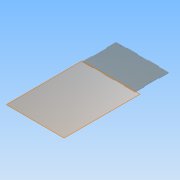
# Autodesk Inventor part: back part
Saved by Autodesk Inventor 2017 (Build 210142000, 142)
## iProperties
Part Number: back part
Material: Типовые
Document SubType Name: Modeling
Designer: Max
Mass: 385.563 g
Surface Area: 1987.62 cm^2
Volume: 385.563 cm^3
Density: 1 g/cm^3
Appearance: Поликарбонат — дымчатый
Author: Max
Autodesk Inventor part; units mm, degrees
(part 1 of 2)
ref_plane "YZ Plane" through (0, 0, 0) normal (1, 0, 0) x (0, 1, 0)
ref_plane "XZ Plane" through (0, 0, 0) normal (0, 1, 0) x (-1, 0, 0)
ref_plane "XY Plane" through (0, 0, 0) normal (0, 0, 1) x (1, 0, 0)
ref_plane "РабПлоскость1" through (0, 0, 0) normal (0, 0, 1) x (1, 0, 0)
sketch "Эскиз1" plane through (0, 0, 0) normal (0, 0, 1) x (1, 0, 0)
  line L0 (1.5, 784) -> (1.5, 779)
  line L1 (1.5, 779) -> (2.8, 779)
  line L2 (2.8, 779) -> (2.8, 776.55)
  line L3 (2.8, 776.55) -> (1.5, 776.55)
  line L4 (1.5, 776.55) -> (1.5, 775.5)
  line L5 (1.5, 775.5) -> (-1.5, 775.5)
  line L6 (-1.5, 775.5) -> (-1.5, 776.55)
  line L7 (-1.5, 776.55) -> (-2.8, 776.55)
  line L8 (-2.8, 776.55) -> (-2.8, 779)
  line L9 (-2.8, 779) -> (-1.5, 779)
  line L10 (-1.5, 779) -> (-1.5, 784)
  line L11 (-1.5, 784) -> (-39.3, 784)
  line L12 (-39.3, 784) -> (-39.3, 788)
  line L13 (-39.3, 788) -> (-116.7, 788)
  line L14 (-116.7, 788) -> (-116.7, 784)
  line L15 (-116.7, 784) -> (-154.35, 784)
  line L16 (-154.35, 784) -> (-154.35, 779)
  line L17 (-154.35, 779) -> (-153.05, 779)
  line L18 (-153.05, 779) -> (-153.05, 776.55)
  line L19 (-153.05, 776.55) -> (-154.35, 776.55)
  line L20 (-154.35, 776.55) -> (-154.35, 775.5)
  line L21 (-154.35, 775.5) -> (-157.35, 775.5)
  line L22 (-157.35, 775.5) -> (-157.35, 776.55)
  line L23 (-157.35, 776.55) -> (-158.65, 776.55)
  line L24 (-158.65, 776.55) -> (-158.65, 779)
  line L25 (-158.65, 779) -> (-157.35, 779)
  line L26 (-157.35, 779) -> (-157.35, 784)
  line L27 (-157.35, 784) -> (-195, 784)
  line L28 (-195, 784) -> (-195, 26) projected
  line L29 (-195, 26) -> (-145, 26) projected
  line L30 (-145, 26) -> (-145, 324) projected
  line L31 (-145, 324) -> (-125, 344) projected
  line L32 (-125, 344) -> (125, 344) projected
  line L33 (125, 344) -> (145, 324) projected
  line L34 (145, 324) -> (145, 26) projected
  line L35 (145, 26) -> (195, 26) projected
  line L36 (195, 26) -> (195, 784) projected
  line L37 (195, 784) -> (157.35, 784)
  line L38 (157.35, 784) -> (157.35, 779)
  line L39 (157.35, 779) -> (158.65, 779)
  line L40 (158.65, 779) -> (158.65, 776.55)
  line L41 (158.65, 776.55) -> (157.35, 776.55)
  line L42 (157.35, 776.55) -> (157.35, 775.5)
  line L43 (157.35, 775.5) -> (154.35, 775.5)
  line L44 (154.35, 775.5) -> (154.35, 776.55)
  line L45 (154.35, 776.55) -> (153.05, 776.55)
  line L46 (153.05, 776.55) -> (153.05, 779)
  line L47 (153.05, 779) -> (154.35, 779)
  line L48 (154.35, 779) -> (154.35, 784)
  line L49 (154.35, 784) -> (116.7, 784)
  line L50 (116.7, 784) -> (116.7, 788)
  line L51 (116.7, 788) -> (39.3, 788)
  line L52 (39.3, 788) -> (39.3, 784)
  line L53 (39.3, 784) -> (1.5, 784)
  circle A0 centre (181, 376) radius 5 projected
  circle A1 centre (-181, 376) radius 5 projected
  circle A2 centre (-179, 349) radius 5 projected
  circle A3 centre (179, 349) radius 5 projected
  line L54 (-131.1498, 477.7505) -> (-131.1498, 487.2505) projected
  arc A4 (-130.8998, 487.5005) -> (-131.1498, 487.2505) centre (-130.8998, 487.2505) ccw projected
  line L55 (-130.8998, 487.5005) -> (-108.8998, 487.5005) projected
  arc A5 (-108.6498, 487.2505) -> (-108.8998, 487.5005) centre (-108.8998, 487.2505) ccw projected
  line L56 (-108.6498, 487.2505) -> (-108.6498, 477.7505) projected
  arc A6 (-108.8998, 477.5005) -> (-108.6498, 477.7505) centre (-108.8998, 477.7505) ccw projected
  line L57 (-108.8998, 477.5005) -> (-130.8998, 477.5005) projected
  arc A7 (-131.1498, 477.7505) -> (-130.8998, 477.5005) centre (-130.8998, 477.7505) ccw projected
  spline S0 degree 2 poles (-108.6858, 451.2309) (-108.6858, 452.7138) (-109.7069, 454.8289) (-110.7523, 455.4245) knots 0 0 0 1 2 2 2 projected
  spline S1 degree 2 poles (-110.7523, 455.4245) (-111.5181, 455.8378) (-113.1955, 455.9229) (-114.3625, 455.9229) knots 0 0 0 1 2 2 2 projected
  line L58 (-114.3625, 455.9229) -> (-118.2036, 455.9229) projected
  line L59 (-118.2036, 455.9229) -> (-118.2036, 458.7187) projected
  line L60 (-118.2036, 458.7187) -> (-113.5602, 458.7187) projected
  spline S2 degree 2 poles (-113.5602, 458.7187) (-111.98, 458.7187) (-109.2207, 458.3176) (-108.0051, 457.5396) knots 0 0 0 1 2 2 2 projected
  spline S3 degree 2 poles (-108.0051, 457.5396) (-106.5343, 456.5915) (-104.8203, 453.3825) (-104.8203, 451.2066) knots 0 0 0 1 2 2 2 projected
  spline S4 degree 2 poles (-104.8203, 451.2066) (-104.8203, 449.1036) (-106.6558, 445.7973) (-108.0537, 444.91) knots 0 0 0 1 2 2 2 projected
  spline S5 degree 2 poles (-108.0537, 444.91) (-109.2206, 444.1563) (-111.9678, 443.7186) (-113.5116, 443.7187) knots 0 0 0 1 2 2 2 projected
  line L61 (-113.5116, 443.7187) -> (-118.2036, 443.7187) projected
  line L62 (-118.2036, 443.7187) -> (-118.2036, 446.5267) projected
  line L63 (-118.2036, 446.5267) -> (-114.3625, 446.5267) projected
  spline S6 degree 2 poles (-114.3625, 446.5267) (-113.0983, 446.5267) (-111.36, 446.6118) (-110.5699, 447.1101) knots 0 0 0 1 2 2 2 projected
  spline S7 degree 2 poles (-110.5699, 447.1101) (-109.6461, 447.6936) (-108.6858, 449.7479) (-108.6858, 451.2309) knots 0 0 0 1 2 2 2 projected
  line L64 (-122.3998, 476.0005) -> (-122.3998, 477.0005) projected
  line L65 (-122.3998, 477.0005) -> (-117.3998, 477.0005) projected
  line L66 (-117.3998, 477.0005) -> (-117.3998, 476.0005) projected
  line L67 (-117.3998, 476.0005) -> (-115.3998, 476.0005) projected
  line L68 (-115.3998, 476.0005) -> (-115.3998, 473.0005) projected
  spline S8 degree 2 poles (-115.3998, 473.0005) (-116.5248, 471.7942) (-117.6498, 473.0005) knots -0.936411 -0.936411 -0.936411 0 0 0 weights 1 1.154701 1 projected
  spline S9 degree 2 poles (-117.6498, 473.0005) (-119.8998, 471.7942) (-122.1498, 473.0005) knots -0.936411 -0.936411 -0.936411 0 0 0 weights 1 1.154701 1 projected
  spline S10 degree 2 poles (-122.1498, 473.0005) (-123.2748, 471.7942) (-124.3998, 473.0005) knots 0 0 0 0.936411 0.936411 0.936411 weights 1 1.154701 1 projected
  line L69 (-124.3998, 473.0005) -> (-124.3998, 476.0005) projected
  line L70 (-124.3998, 476.0005) -> (-122.3998, 476.0005) projected
  line L71 (-119.5248, 468.5774) -> (-120.2748, 468.5774) projected
  line L72 (-120.2748, 468.5774) -> (-123.3048, 471.8264) projected
  spline S11 degree 3 poles (-123.3048, 471.8264) (-123.2674, 471.8256) (-123.1923, 471.8269) (-123.099, 471.836) (-123.0063, 471.8503) (-122.9329, 471.866) (-122.8423, 471.8907) (-122.7708, 471.9142) (-122.6828, 471.9483) (-122.6134, 471.9792) (-122.528, 472.0219) (-122.4606, 472.0595) (-122.3773, 472.1105) (-122.3114, 472.1544) (-122.2297, 472.2133) (-122.1486, 472.2762) (-122.0839, 472.3308) (-122.0515, 472.3592) knots 0.459691 0.459691 0.459691 0.459691 0.491589 0.523488 0.539437 0.571336 0.587285 0.619184 0.635133 0.667032 0.682981 0.71488 0.730829 0.762728 0.778677 0.810576 0.842474 0.842474 0.842474 0.842474 projected
  spline S12 degree 3 poles (-122.0515, 472.3592) (-121.923, 472.2982) (-121.6714, 472.1878) (-121.3667, 472.0767) (-121.0671, 471.9849) (-120.8308, 471.9266) (-120.538, 471.872) (-120.3054, 471.843) (-120.0156, 471.8248) (-119.7841, 471.8248) (-119.4942, 471.843) (-119.2616, 471.872) (-118.9103, 471.9375) (-118.4363, 472.064) (-118.0051, 472.2371) (-117.7481, 472.3592) knots 0.060134 0.060134 0.060134 0.060134 0.128146 0.196158 0.230164 0.298176 0.332182 0.400194 0.4342 0.502211 0.536217 0.604229 0.638235 0.740253 0.876277 0.876277 0.876277 0.876277 projected
  spline S13 degree 3 poles (-117.7481, 472.3592) (-117.7158, 472.3308) (-117.6511, 472.2762) (-117.5699, 472.2133) (-117.4882, 472.1544) (-117.4223, 472.1105) (-117.3391, 472.0595) (-117.2717, 472.0219) (-117.1862, 471.9792) (-117.1169, 471.9483) (-117.0288, 471.9142) (-116.9573, 471.8907) (-116.8667, 471.866) (-116.7933, 471.8503) (-116.7007, 471.836) (-116.6073, 471.8269) (-116.5323, 471.8256) (-116.4948, 471.8264) knots 0.093937 0.093937 0.093937 0.093937 0.125835 0.157734 0.173683 0.205582 0.221531 0.25343 0.269379 0.301278 0.317227 0.349126 0.365075 0.396974 0.412923 0.444822 0.47672 0.47672 0.47672 0.47672 projected
  line L73 (-116.4948, 471.8264) -> (-119.5248, 468.5774) projected
  line L74 (-114.4354, 446.5678) -> (-118.2036, 446.5678) projected
  line L75 (-118.2036, 446.5678) -> (-118.2036, 455.9186) projected
  line L76 (-118.2036, 455.9186) -> (-114.4354, 455.9186) projected
  line L77 (-114.4354, 455.9186) -> (-114.4354, 446.5678) projected
  arc A8 (-119.3998, 461.3273) -> (-120.8998, 462.8273) centre (-120.8998, 461.3273) ccw projected
  line L78 (-119.3998, 461.3273) -> (-119.3998, 460.8273) projected
  line L79 (-119.3998, 460.8273) -> (-120.3998, 460.8273) projected
  line L80 (-120.3998, 460.8273) -> (-120.3998, 461.3273) projected
  arc A9 (-120.3998, 461.3273) -> (-120.8998, 461.8273) centre (-120.8998, 461.3273) ccw projected
  line L81 (-120.8998, 461.8273) -> (-127.3998, 461.8273) projected
  arc A10 (-127.3998, 464.8273) -> (-127.3998, 461.8273) centre (-127.3998, 463.3273) ccw projected
  line L82 (-127.3998, 464.8273) -> (-112.3998, 464.8273) projected
  arc A11 (-112.3998, 464.8273) -> (-112.3998, 465.8273) centre (-112.3998, 465.3273) ccw projected
  line L83 (-112.3998, 465.8273) -> (-118.8998, 465.8273) projected
  arc A12 (-120.3998, 467.3273) -> (-118.8998, 465.8273) centre (-118.8998, 467.3273) ccw projected
  line L84 (-120.3998, 467.3273) -> (-120.3998, 467.8273) projected
  line L85 (-120.3998, 467.8273) -> (-119.3998, 467.8273) projected
  line L86 (-119.3998, 467.8273) -> (-119.3998, 467.3273) projected
  arc A13 (-119.3998, 467.3273) -> (-118.8998, 466.8273) centre (-118.8998, 467.3273) ccw projected
  line L87 (-118.8998, 466.8273) -> (-112.3998, 466.8273) projected
  arc A14 (-112.3998, 463.8273) -> (-112.3998, 466.8273) centre (-112.3998, 465.3273) ccw projected
  line L88 (-112.3998, 463.8273) -> (-127.3998, 463.8273) projected
  arc A15 (-127.3998, 463.8273) -> (-127.3998, 462.8273) centre (-127.3998, 463.3273) ccw projected
  line L89 (-127.3998, 462.8273) -> (-120.8998, 462.8273) projected
  spline S14 degree 2 poles (-122.6526, 458.1231) (-121.8868, 457.649) (-121.121, 456.1904) (-121.121, 455.2787) knots 0 0 0 1 2 2 2 projected
  spline S15 degree 2 poles (-121.121, 455.2787) (-121.121, 453.9902) (-122.604, 452.0696) (-123.8195, 451.79) knots 0 0 0 1 2 2 2 projected
  line L90 (-123.8195, 451.79) -> (-123.8195, 451.6442) projected
  spline S16 degree 2 poles (-123.8195, 451.6442) (-123.2847, 451.5712) (-122.2636, 451.1822) (-121.7774, 450.7446) knots 0 0 0 1 2 2 2 projected
  spline S17 degree 2 poles (-121.7774, 450.7446) (-121.3276, 450.3557) (-120.732, 449.1158) (-120.732, 448.2649) knots 0 0 0 1 2 2 2 projected
  spline S18 degree 2 poles (-120.732, 448.2649) (-120.732, 447.1587) (-121.5464, 445.3476) (-122.3365, 444.7155) knots 0 0 0 1 2 2 2 projected
  spline S19 degree 2 poles (-122.3365, 444.7155) (-123.1267, 444.0834) (-125.2782, 443.4027) (-126.822, 443.4027) knots 0 0 0 1 2 2 2 projected
  spline S20 degree 2 poles (-126.822, 443.4027) (-128.5724, 443.4026) (-131.0764, 443.9861) (-131.8665, 444.3508) knots 0 0 0 1 2 2 2 projected
  line L91 (-131.8665, 444.3508) -> (-131.8665, 447.6085) projected
  line L92 (-131.8665, 447.6085) -> (-131.5019, 447.6085) projected
  spline S21 degree 2 poles (-131.5019, 447.6085) (-130.6753, 447.0858) (-128.4508, 446.3079) (-127.527, 446.3079) knots 0 0 0 1 2 2 2 projected
  spline S22 degree 2 poles (-127.527, 446.3079) (-126.98, 446.3079) (-125.7036, 446.5024) (-125.266, 446.8184) knots 0 0 0 1 2 2 2 projected
  spline S23 degree 2 poles (-125.266, 446.8184) (-124.9257, 447.0737) (-124.5124, 447.8151) (-124.5124, 448.4837) knots 0 0 0 1 2 2 2 projected
  spline S24 degree 2 poles (-124.5124, 448.4837) (-124.5124, 449.1523) (-125.0959, 449.8694) (-125.5821, 450.0396) knots 0 0 0 1 2 2 2 projected
  spline S25 degree 2 poles (-125.5821, 450.0396) (-126.0683, 450.2098) (-127.4176, 450.2463) (-127.9403, 450.2463) knots 0 0 0 1 2 2 2 projected
  line L93 (-127.9403, 450.2463) -> (-128.5845, 450.2463) projected
  line L94 (-128.5845, 450.2463) -> (-128.5845, 452.884) projected
  line L95 (-128.5845, 452.884) -> (-127.9889, 452.884) projected
  spline S26 degree 2 poles (-127.9889, 452.884) (-127.3082, 452.884) (-126.1534, 453.0056) (-125.7523, 453.1879) knots 0 0 0 1 2 2 2 projected
  spline S27 degree 2 poles (-125.7523, 453.1879) (-125.3511, 453.3824) (-124.9014, 454.0631) (-124.9014, 454.6466) knots 0 0 0 1 2 2 2 projected
  spline S28 degree 2 poles (-124.9014, 454.6466) (-124.9014, 455.1085) (-125.3268, 455.6798) (-125.6307, 455.8378) knots 0 0 0 1 2 2 2 projected
  spline S29 degree 2 poles (-125.6307, 455.8378) (-125.9954, 456.0202) (-126.9678, 456.1417) (-127.3082, 456.1417) knots 0 0 0 1 2 2 2 projected
  spline S30 degree 2 poles (-127.3082, 456.1417) (-127.8552, 456.1417) (-129.01, 455.8864) (-129.5448, 455.6798) knots 0 0 0 1 2 2 2 projected
  spline S31 degree 2 poles (-129.5448, 455.6798) (-129.9703, 455.5218) (-130.7084, 455.1139) (-130.8976, 455.0047) knots 0 0 0 1 1.597943 1.597943 1.597943 projected
  line L96 (-130.8976, 455.0047) -> (-131.3629, 454.8775) projected
  line L97 (-131.3629, 454.8775) -> (-131.4289, 454.8775) projected
  line L98 (-131.4289, 454.8775) -> (-131.4289, 458.0866) projected
  spline S32 degree 2 poles (-131.4289, 458.0866) (-130.651, 458.4148) (-128.0254, 459.0348) (-126.6518, 459.0348) knots 0 0 0 1 2 2 2 projected
  spline S33 degree 2 poles (-126.6518, 459.0348) (-125.3147, 459.0348) (-123.3455, 458.5729) (-122.6526, 458.1231) knots 0 0 0 1 2 2 2 projected
  line L99 (-119.9951, 430.5006) -> (-119.9951, 437.0006) projected
  arc A16 (-119.9951, 437.0006) -> (-119.9952, 437.0006) centre (-119.8998, 464.5005) ccw projected
  line L100 (-119.9952, 437.0006) -> (-119.9952, 430.5006) projected
  arc A17 (-124.3998, 430.7996) -> (-119.9952, 430.5006) centre (-119.8998, 464.5005) ccw projected
  arc A18 (-126.1498, 434.137) -> (-124.3998, 430.7996) centre (-112.6193, 439.1042) ccw projected
  arc A19 (-136.9506, 438.6109) -> (-126.1498, 434.137) centre (-119.8998, 464.5005) ccw projected
  arc A20 (-140.548, 437.4884) -> (-136.9506, 438.6109) centre (-143.0058, 451.6907) ccw projected
  arc A21 (-146.9119, 443.8523) -> (-140.548, 437.4884) centre (-119.8998, 464.5005) ccw projected
  arc A22 (-145.7894, 447.4497) -> (-146.9119, 443.8523) centre (-132.7096, 441.3945) ccw projected
  arc A23 (-150.2632, 458.2505) -> (-145.7894, 447.4497) centre (-119.8998, 464.5005) ccw projected
  arc A24 (-153.6007, 460.0005) -> (-150.2632, 458.2505) centre (-145.2961, 471.781) ccw projected
  arc A25 (-153.6007, 469.0005) -> (-153.6007, 460.0005) centre (-119.8998, 464.5005) ccw projected
  arc A26 (-150.2632, 470.7505) -> (-153.6007, 469.0005) centre (-145.2961, 457.2199) ccw projected
  arc A27 (-145.7894, 481.5512) -> (-150.2632, 470.7505) centre (-119.8998, 464.5005) ccw projected
  arc A28 (-146.9119, 485.1486) -> (-145.7894, 481.5512) centre (-132.7096, 487.6064) ccw projected
  arc A29 (-140.548, 491.5126) -> (-146.9119, 485.1486) centre (-119.8998, 464.5005) ccw projected
  arc A30 (-136.9506, 490.3901) -> (-140.548, 491.5126) centre (-143.0058, 477.3102) ccw projected
  arc A31 (-126.1498, 494.8639) -> (-136.9506, 490.3901) centre (-119.8998, 464.5005) ccw projected
  arc A32 (-124.3998, 498.2014) -> (-126.1498, 494.8639) centre (-112.6193, 489.8967) ccw projected
  arc A33 (-115.3998, 498.2014) -> (-124.3998, 498.2014) centre (-119.8998, 464.5005) ccw projected
  arc A34 (-113.6498, 494.8639) -> (-115.3998, 498.2014) centre (-127.1803, 489.8967) ccw projected
  arc A35 (-102.8491, 490.3901) -> (-113.6498, 494.8639) centre (-119.8998, 464.5005) ccw projected
  arc A36 (-99.2517, 491.5126) -> (-102.8491, 490.3901) centre (-96.7939, 477.3102) ccw projected
  arc A37 (-92.8877, 485.1486) -> (-99.2517, 491.5126) centre (-119.8998, 464.5005) ccw projected
  arc A38 (-94.0102, 481.5512) -> (-92.8877, 485.1486) centre (-107.0901, 487.6064) ccw projected
  arc A39 (-89.5364, 470.7505) -> (-94.0102, 481.5512) centre (-119.8998, 464.5005) ccw projected
  arc A40 (-86.1989, 469.0005) -> (-89.5364, 470.7505) centre (-94.5036, 457.2199) ccw projected
  arc A41 (-86.1989, 460.0005) -> (-86.1989, 469.0005) centre (-119.8998, 464.5005) ccw projected
  arc A42 (-89.5364, 458.2505) -> (-86.1989, 460.0005) centre (-94.5036, 471.781) ccw projected
  arc A43 (-94.0102, 447.4497) -> (-89.5364, 458.2505) centre (-119.8998, 464.5005) ccw projected
  arc A44 (-92.8877, 443.8523) -> (-94.0102, 447.4497) centre (-107.0901, 441.3945) ccw projected
  arc A45 (-99.2517, 437.4884) -> (-92.8877, 443.8523) centre (-119.8998, 464.5005) ccw projected
  arc A46 (-102.8491, 438.6109) -> (-99.2517, 437.4884) centre (-96.7939, 451.6907) ccw projected
  arc A47 (-113.6498, 434.137) -> (-102.8491, 438.6109) centre (-119.8998, 464.5005) ccw projected
  arc A48 (-115.3998, 430.7996) -> (-113.6498, 434.137) centre (-127.1803, 439.1042) ccw projected
  arc A49 (-119.9951, 430.5006) -> (-115.3998, 430.7996) centre (-119.8998, 464.5005) ccw projected
  circle A50 centre (1, 464) radius 20.6 projected
  circle A51 centre (179.5, 40) radius 2 projected
  circle A52 centre (-179.5, 79.5) radius 2 projected
  circle A53 centre (-179.5, 337) radius 2 projected
  circle A54 centre (179.5, 337) radius 2 projected
  circle A55 centre (179.5, 255) radius 2.875 projected
  circle A56 centre (-179.5, 308) radius 2 projected
  circle A57 centre (-179.5, 40) radius 2 projected
  circle A58 centre (-158.75, 122) radius 1.5 projected
  circle A59 centre (-158.75, 254) radius 1.5 projected
  circle A60 centre (-158.75, 284) radius 1.5 projected
  circle A61 centre (-158.75, 92) radius 1.5 projected
  circle A62 centre (150.2671, 178.4783) radius 1.5 projected
  line L101 (116.2244, 383.4424) -> (116.2244, 380.5646) projected
  line L102 (116.2244, 380.5646) -> (110.4314, 380.5646) projected
  line L103 (110.4314, 380.5646) -> (110.1311, 378.6127) projected
  spline S34 degree 2 poles (110.1311, 378.6127) (110.7316, 378.888) (111.9078, 379.1758) (112.4833, 379.1758) knots 0 0 0 1 2 2 2 projected
  spline S35 degree 2 poles (112.4833, 379.1758) (114.4227, 379.1758) (116.85, 376.811) (116.85, 375.0218) knots 0 0 0 1 2 2 2 projected
  spline S36 degree 2 poles (116.85, 375.0218) (116.85, 373.7706) (115.5988, 371.4433) (113.3091, 370.2172) (111.5199, 370.2172) knots 0 0 0 1 2 3 3 3 projected
  spline S37 degree 2 poles (111.5199, 370.2172) (110.2312, 370.2172) (108.4044, 370.7051) (107.1157, 371.6686) (106.3149, 372.8947) (106.0521, 373.8081) knots 0 0 0 1 2 3 4 4 4 projected
  line L104 (106.0521, 373.8081) -> (109.7057, 374.2085) projected
  spline S38 degree 2 poles (109.7057, 374.2085) (109.8433, 373.3327) (110.8067, 372.4193) (111.4824, 372.4193) knots 0 0 0 1 2 2 2 projected
  spline S39 degree 2 poles (111.4824, 372.4193) (112.2331, 372.4193) (113.209, 373.5579) (113.209, 374.6965) knots 0 0 0 1 2 2 2 projected
  spline S40 degree 2 poles (113.209, 374.6965) (113.209, 375.8601) (112.2206, 376.9361) (111.4073, 376.9361) knots 0 0 0 1 2 2 2 projected
  spline S41 degree 2 poles (111.4073, 376.9361) (110.8818, 376.9361) (110.3938, 376.6734) knots 0 0 0 1 1 1 projected
  spline S42 degree 2 poles (110.3938, 376.6734) (110.0435, 376.4982) (109.6056, 376.0102) knots 0 0 0 1 1 1 projected
  line L105 (109.6056, 376.0102) -> (106.5276, 376.4481) projected
  line L106 (106.5276, 376.4481) -> (107.6662, 383.4424) projected
  line L107 (107.6662, 383.4424) -> (116.2244, 383.4424) projected
  spline S43 degree 2 poles (77.5998, 374.9842) (77.7249, 374.0458) (78.1003, 373.5579) knots 0 0 0 1 1 1 projected
  spline S44 degree 2 poles (78.1003, 373.5579) (78.7259, 372.7696) (79.8895, 372.7696) knots 0 0 0 1 1 1 projected
  spline S45 degree 2 poles (79.8895, 372.7696) (80.7403, 372.7696) (81.6787, 373.5829) (81.6787, 374.1084) knots 0 0 0 1 2 2 2 projected
  spline S46 degree 2 poles (81.6787, 374.1084) (81.6787, 374.6089) (81.2283, 375.0093) knots 0 0 0 1 1 1 projected
  spline S47 degree 2 poles (81.2283, 375.0093) (80.7904, 375.4096) (79.1763, 375.7725) knots 0 0 0 1 1 1 projected
  spline S48 degree 2 poles (79.1763, 375.7725) (76.5237, 376.3606) (75.3977, 377.349) knots 0 0 0 1 1 1 projected
  spline S49 degree 2 poles (75.3977, 377.349) (74.2591, 378.3375) (74.2591, 379.8639) knots 0 0 0 1 1 1 projected
  spline S50 degree 2 poles (74.2591, 379.8639) (74.2591, 380.8649) (75.4227, 382.6416) (77.7624, 383.6676) (79.7894, 383.6676) knots 0 0 0 1 2 3 3 3 projected
  spline S51 degree 2 poles (79.7894, 383.6676) (82.2918, 383.6676) (84.9068, 381.8158) (85.157, 379.7889) knots 0 0 0 1 2 2 2 projected
  line L108 (85.157, 379.7889) -> (81.3659, 379.5636) projected
  spline S52 degree 2 poles (81.3659, 379.5636) (81.2158, 380.4395) (80.2398, 381.2403) (79.389, 381.2403) knots 0 0 0 1 2 2 2 projected
  spline S53 degree 2 poles (79.389, 381.2403) (78.6883, 381.2403) (77.9751, 380.6522) (77.9751, 380.2143) knots 0 0 0 1 2 2 2 projected
  spline S54 degree 2 poles (77.9751, 380.2143) (77.9751, 379.914) (78.2754, 379.6637) knots 0 0 0 1 1 1 projected
  spline S55 degree 2 poles (78.2754, 379.6637) (78.5632, 379.401) (79.6267, 379.1883) knots 0 0 0 1 1 1 projected
  spline S56 degree 2 poles (79.6267, 379.1883) (82.2668, 378.6127) (84.544, 377.4491) (85.5825, 375.735) (85.5825, 374.6714) knots 0 0 0 1 2 3 3 3 projected
  spline S57 degree 2 poles (85.5825, 374.6714) (85.5825, 373.4202) (84.1936, 371.3057) (81.7162, 370.2172) (79.8144, 370.2172) knots 0 0 0 1 2 3 3 3 projected
  spline S58 degree 2 poles (79.8144, 370.2172) (76.4987, 370.2172) (73.9338, 372.7696) (73.7711, 374.7465) knots 0 0 0 1 2 2 2 projected
  line L109 (73.7711, 374.7465) -> (77.5998, 374.9842) projected
  spline S59 degree 2 poles (65.5507, 383.6676) (68.7913, 383.6676) (72.3072, 380.1767) (72.3072, 377.0362) knots 0 0 0 1 2 2 2 projected
  spline S60 degree 2 poles (72.3072, 377.0362) (72.3072, 374.759) (70.7682, 371.8437) (67.8654, 370.2172) (65.7008, 370.2172) knots 0 0 0 1 2 3 3 3 projected
  spline S61 degree 2 poles (65.7008, 370.2172) (63.5112, 370.2172) (60.621, 371.6185) (58.8317, 374.6589) (58.8317, 376.9361) knots 0 0 0 1 2 3 3 3 projected
  spline S62 degree 2 poles (58.8317, 376.9361) (58.8317, 380.1142) (62.3852, 383.6676) (65.5507, 383.6676) knots 0 0 0 1 2 2 2 projected
  line L110 (35.6094, 377.8495) -> (41.8154, 377.8495) projected
  line L111 (41.8154, 377.8495) -> (41.8154, 372.3192) projected
  spline S63 degree 2 poles (41.8154, 372.3192) (40.0262, 371.093) (37.286, 370.2172) (35.4092, 370.2172) knots 0 0 0 1 2 2 2 projected
  spline S64 degree 2 poles (35.4092, 370.2172) (33.0945, 370.2172) (30.1667, 371.7937) (28.5651, 374.9217) (28.5651, 376.9486) knots 0 0 0 1 2 3 3 3 projected
  spline S65 degree 2 poles (28.5651, 376.9486) (28.5651, 379.0757) (30.3168, 382.2162) (32.0185, 383.042) knots 0 0 0 1 2 2 2 projected
  spline S66 degree 2 poles (32.0185, 383.042) (33.3447, 383.6676) (35.5719, 383.6676) knots 0 0 0 1 1 1 projected
  spline S67 degree 2 poles (35.5719, 383.6676) (37.7365, 383.6676) (39.876, 382.8918) (41.2899, 381.2403) (41.6402, 379.9891) knots 0 0 0 1 2 3 3 3 projected
  line L112 (41.6402, 379.9891) -> (37.7615, 379.2884) projected
  spline S68 degree 2 poles (37.7615, 379.2884) (37.5238, 380.0266) (36.3726, 380.8148) (35.4843, 380.8148) knots 0 0 0 1 2 2 2 projected
  spline S69 degree 2 poles (35.4843, 380.8148) (34.1705, 380.8148) (32.594, 378.9756) (32.594, 376.9862) knots 0 0 0 1 2 2 2 projected
  spline S70 degree 2 poles (32.594, 376.9862) (32.594, 374.8841) (34.183, 373.0699) (35.6094, 373.0699) knots 0 0 0 1 2 2 2 projected
  spline S71 degree 2 poles (35.6094, 373.0699) (36.2851, 373.0699) (37.5112, 373.4578) (38.2995, 373.9332) knots 0 0 0 1 2 2 2 projected
  line L113 (38.2995, 373.9332) -> (38.2995, 375.1469) projected
  line L114 (38.2995, 375.1469) -> (35.6094, 375.1469) projected
  line L115 (35.6094, 375.1469) -> (35.6094, 377.8495) projected
  line L116 (8.9212, 383.4424) -> (15.6152, 383.4424) projected
  spline S72 degree 2 poles (15.6152, 383.4424) (17.467, 383.4424) (19.4439, 382.8043) (20.645, 381.0776) (20.645, 379.8389) knots 0 0 0 1 2 3 3 3 projected
  spline S73 degree 2 poles (20.645, 379.8389) (20.645, 378.7504) (19.7191, 377.1864) (18.9184, 376.6984) knots 0 0 0 1 2 2 2 projected
  spline S74 degree 2 poles (18.9184, 376.6984) (18.4054, 376.3856) (17.5045, 376.1854) knots 0 0 0 1 1 1 projected
  spline S75 degree 2 poles (17.5045, 376.1854) (18.2177, 375.9477) (18.5555, 375.7099) knots 0 0 0 1 1 1 projected
  spline S76 degree 2 poles (18.5555, 375.7099) (18.7682, 375.5473) (19.6065, 374.4963) (19.7567, 374.2085) knots 0 0 0 1 2 2 2 projected
  line L117 (19.7567, 374.2085) -> (21.696, 370.4424) projected
  line L118 (21.696, 370.4424) -> (17.1542, 370.4424) projected
  line L119 (17.1542, 370.4424) -> (15.0146, 374.4212) projected
  spline S77 degree 2 poles (15.0146, 374.4212) (14.6142, 375.1844) (14.3014, 375.4222) knots 0 0 0 1 1 1 projected
  spline S78 degree 2 poles (14.3014, 375.4222) (13.8635, 375.7225) (13.313, 375.7225) knots 0 0 0 1 1 1 projected
  line L120 (13.313, 375.7225) -> (12.9626, 375.7225) projected
  line L121 (12.9626, 375.7225) -> (12.9626, 370.4424) projected
  line L122 (12.9626, 370.4424) -> (8.9212, 370.4424) projected
  line L123 (8.9212, 370.4424) -> (8.9212, 383.4424) projected
  line L124 (-1.8516, 372.5944) -> (-2.4897, 370.4424) projected
  line L125 (-2.4897, 370.4424) -> (-6.5937, 370.4424) projected
  line L126 (-6.5937, 370.4424) -> (-1.7015, 383.4424) projected
  line L127 (-1.7015, 383.4424) -> (2.6903, 383.4424) projected
  line L128 (2.6903, 383.4424) -> (7.5699, 370.4424) projected
  line L129 (7.5699, 370.4424) -> (3.3659, 370.4424) projected
  line L130 (3.3659, 370.4424) -> (2.7153, 372.5944) projected
  line L131 (2.7153, 372.5944) -> (-1.8516, 372.5944) projected
  spline S79 degree 2 poles (-25.0114, 383.4424) (-23.1346, 383.4424) (-21.1201, 381.5781) (-21.1201, 380.2018) knots 0 0 0 1 2 2 2 projected
  spline S80 degree 2 poles (-21.1201, 380.2018) (-21.1201, 379.0507) (-21.8333, 378.2249) knots 0 0 0 1 1 1 projected
  spline S81 degree 2 poles (-21.8333, 378.2249) (-22.3213, 377.6743) (-23.2472, 377.349) knots 0 0 0 1 1 1 projected
  spline S82 degree 2 poles (-23.2472, 377.349) (-21.8458, 377.0112) (-20.5196, 375.3721) (-20.5196, 374.1334) knots 0 0 0 1 2 2 2 projected
  spline S83 degree 2 poles (-20.5196, 374.1334) (-20.5196, 373.1325) (-21.458, 371.5184) (-22.2712, 371.043) knots 0 0 0 1 2 2 2 projected
  spline S84 degree 2 poles (-22.2712, 371.043) (-22.7842, 370.7552) (-23.7977, 370.6175) knots 0 0 0 1 1 1 projected
  spline S85 degree 2 poles (-23.7977, 370.6175) (-25.1615, 370.4424) (-25.5994, 370.4424) knots 0 0 0 1 1 1 projected
  line L132 (-25.5994, 370.4424) -> (-32.5311, 370.4424) projected
  line L133 (-32.5311, 370.4424) -> (-32.5311, 383.4424) projected
  line L134 (-32.5311, 383.4424) -> (-25.0114, 383.4424) projected
  line L135 (-65.0999, 383.4424) -> (-60.1952, 376.248) projected
  line L136 (-60.1952, 376.248) -> (-60.1952, 383.4424) projected
  line L137 (-60.1952, 383.4424) -> (-56.4041, 383.4424) projected
  line L138 (-56.4041, 383.4424) -> (-56.4041, 370.4424) projected
  line L139 (-56.4041, 370.4424) -> (-60.1952, 370.4424) projected
  line L140 (-60.1952, 370.4424) -> (-65.0749, 377.5993) projected
  line L141 (-65.0749, 377.5993) -> (-65.0749, 370.4424) projected
  line L142 (-65.0749, 370.4424) -> (-68.8535, 370.4424) projected
  line L143 (-68.8535, 370.4424) -> (-68.8535, 383.4424) projected
  line L144 (-68.8535, 383.4424) -> (-65.0999, 383.4424) projected
  line L145 (-86.9334, 383.4424) -> (-84.3184, 379.0632) projected
  line L146 (-84.3184, 379.0632) -> (-81.6909, 383.4424) projected
  line L147 (-81.6909, 383.4424) -> (-77.2491, 383.4424) projected
  line L148 (-77.2491, 383.4424) -> (-82.304, 375.8851) projected
  line L149 (-82.304, 375.8851) -> (-82.304, 370.4424) projected
  line L150 (-82.304, 370.4424) -> (-86.3328, 370.4424) projected
  line L151 (-86.3328, 370.4424) -> (-86.3328, 375.8851) projected
  line L152 (-86.3328, 375.8851) -> (-91.4002, 383.4424) projected
  line L153 (-91.4002, 383.4424) -> (-86.9334, 383.4424) projected
  line L154 (-104.3877, 383.4424) -> (-104.3877, 380.6522) projected
  line L155 (-104.3877, 380.6522) -> (-110.2684, 380.6522) projected
  line L156 (-110.2684, 380.6522) -> (-110.2684, 378.3875) projected
  line L157 (-110.2684, 378.3875) -> (-105.251, 378.3875) projected
  line L158 (-105.251, 378.3875) -> (-105.251, 375.76) projected
  line L159 (-105.251, 375.76) -> (-110.2684, 375.76) projected
  line L160 (-110.2684, 375.76) -> (-110.2684, 370.4424) projected
  line L161 (-110.2684, 370.4424) -> (-114.3097, 370.4424) projected
  line L162 (-114.3097, 370.4424) -> (-114.3097, 383.4424) projected
  line L163 (-114.3097, 383.4424) -> (-104.3877, 383.4424) projected
  line L164 (-98.1942, 383.4424) -> (-98.1942, 373.6455) projected
  line L165 (-98.1942, 373.6455) -> (-91.9257, 373.6455) projected
  line L166 (-91.9257, 373.6455) -> (-91.9257, 370.4424) projected
  line L167 (-91.9257, 370.4424) -> (-102.2106, 370.4424) projected
  line L168 (-102.2106, 370.4424) -> (-102.2106, 383.4424) projected
  line L169 (-102.2106, 383.4424) -> (-98.1942, 383.4424) projected
  line L170 (-71.7563, 383.4424) -> (-71.7563, 370.4424) projected
  line L171 (-71.7563, 370.4424) -> (-75.7852, 370.4424) projected
  line L172 (-75.7852, 370.4424) -> (-75.7852, 383.4424) projected
  line L173 (-75.7852, 383.4424) -> (-71.7563, 383.4424) projected
  line L174 (-47.1827, 377.8495) -> (-40.9767, 377.8495) projected
  line L175 (-40.9767, 377.8495) -> (-40.9767, 372.3192) projected
  spline S86 degree 2 poles (-40.9767, 372.3192) (-42.7659, 371.093) (-45.5061, 370.2172) (-47.3829, 370.2172) knots 0 0 0 1 2 2 2 projected
  spline S87 degree 2 poles (-47.3829, 370.2172) (-49.6976, 370.2172) (-52.6254, 371.7937) (-54.227, 374.9217) (-54.227, 376.9486) knots 0 0 0 1 2 3 3 3 projected
  spline S88 degree 2 poles (-54.227, 376.9486) (-54.227, 379.0757) (-52.4753, 382.2162) (-50.7736, 383.042) knots 0 0 0 1 2 2 2 projected
  spline S89 degree 2 poles (-50.7736, 383.042) (-49.4474, 383.6676) (-47.2202, 383.6676) knots 0 0 0 1 1 1 projected
  spline S90 degree 2 poles (-47.2202, 383.6676) (-45.0557, 383.6676) (-42.9161, 382.8918) (-41.5022, 381.2403) (-41.1519, 379.9891) knots 0 0 0 1 2 3 3 3 projected
  line L176 (-41.1519, 379.9891) -> (-45.0306, 379.2884) projected
  spline S91 degree 2 poles (-45.0306, 379.2884) (-45.2684, 380.0266) (-46.4195, 380.8148) (-47.3078, 380.8148) knots 0 0 0 1 2 2 2 projected
  spline S92 degree 2 poles (-47.3078, 380.8148) (-48.6216, 380.8148) (-50.1981, 378.9756) (-50.1981, 376.9862) knots 0 0 0 1 2 2 2 projected
  spline S93 degree 2 poles (-50.1981, 376.9862) (-50.1981, 374.8841) (-48.6091, 373.0699) (-47.1827, 373.0699) knots 0 0 0 1 2 2 2 projected
  spline S94 degree 2 poles (-47.1827, 373.0699) (-46.507, 373.0699) (-45.2809, 373.4578) (-44.4926, 373.9332) knots 0 0 0 1 2 2 2 projected
  line L177 (-44.4926, 373.9332) -> (-44.4926, 375.1469) projected
  line L178 (-44.4926, 375.1469) -> (-47.1827, 375.1469) projected
  line L179 (-47.1827, 375.1469) -> (-47.1827, 377.8495) projected
  line L180 (-7.6447, 383.4424) -> (-7.6447, 380.6647) projected
  line L181 (-7.6447, 380.6647) -> (-14.3762, 380.6647) projected
  line L182 (-14.3762, 380.6647) -> (-14.3762, 378.6002) projected
  line L183 (-14.3762, 378.6002) -> (-8.1326, 378.6002) projected
  line L184 (-8.1326, 378.6002) -> (-8.1326, 375.9477) projected
  line L185 (-8.1326, 375.9477) -> (-14.3762, 375.9477) projected
  line L186 (-14.3762, 375.9477) -> (-14.3762, 373.3827) projected
  line L187 (-14.3762, 373.3827) -> (-7.4445, 373.3827) projected
  line L188 (-7.4445, 373.3827) -> (-7.4445, 370.4424) projected
  line L189 (-7.4445, 370.4424) -> (-18.405, 370.4424) projected
  line L190 (-18.405, 370.4424) -> (-18.405, 383.4424) projected
  line L191 (-18.405, 383.4424) -> (-7.6447, 383.4424) projected
  line L192 (48.234, 383.4424) -> (48.234, 378.888) projected
  line L193 (48.234, 378.888) -> (52.6258, 378.888) projected
  line L194 (52.6258, 378.888) -> (52.6258, 383.4424) projected
  line L195 (52.6258, 383.4424) -> (56.6672, 383.4424) projected
  line L196 (56.6672, 383.4424) -> (56.6672, 370.4424) projected
  line L197 (56.6672, 370.4424) -> (52.6258, 370.4424) projected
  line L198 (52.6258, 370.4424) -> (52.6258, 375.6974) projected
  line L199 (52.6258, 375.6974) -> (48.234, 375.6974) projected
  line L200 (48.234, 375.6974) -> (48.234, 370.4424) projected
  line L201 (48.234, 370.4424) -> (44.2177, 370.4424) projected
  line L202 (44.2177, 370.4424) -> (44.2177, 383.4424) projected
  line L203 (44.2177, 383.4424) -> (48.234, 383.4424) projected
  line L204 (98.9078, 383.4424) -> (98.9078, 380.2268) projected
  line L205 (98.9078, 380.2268) -> (94.8038, 380.2268) projected
  line L206 (94.8038, 380.2268) -> (94.8038, 370.4424) projected
  line L207 (94.8038, 370.4424) -> (90.7875, 370.4424) projected
  line L208 (90.7875, 370.4424) -> (90.7875, 380.2268) projected
  line L209 (90.7875, 380.2268) -> (86.6835, 380.2268) projected
  line L210 (86.6835, 380.2268) -> (86.6835, 383.4424) projected
  line L211 (86.6835, 383.4424) -> (98.9078, 383.4424) projected
  line L212 (1.5, 534) -> (1.5, 529) projected
  line L213 (1.5, 529) -> (2.8, 529) projected
  line L214 (2.8, 529) -> (2.8, 526.55) projected
  line L215 (2.8, 526.55) -> (1.5, 526.55) projected
  line L216 (1.5, 526.55) -> (1.5, 525.5) projected
  line L217 (1.5, 525.5) -> (-1.5, 525.5) projected
  line L218 (-1.5, 525.5) -> (-1.5, 526.55) projected
  line L219 (-1.5, 526.55) -> (-2.8, 526.55) projected
  line L220 (-2.8, 526.55) -> (-2.8, 529) projected
  line L221 (-2.8, 529) -> (-1.5, 529) projected
  line L222 (-1.5, 529) -> (-1.5, 534) projected
  line L223 (-1.5, 534) -> (-39.3, 534) projected
  line L224 (-39.3, 534) -> (-39.3, 538) projected
  line L225 (-39.3, 538) -> (-116.7, 538) projected
  line L226 (-116.7, 538) -> (-116.7, 534) projected
  line L227 (-116.7, 534) -> (-154.35, 534) projected
  line L228 (-154.35, 534) -> (-154.35, 529) projected
  line L229 (-154.35, 529) -> (-153.05, 529) projected
  line L230 (-153.05, 529) -> (-153.05, 526.55) projected
  line L231 (-153.05, 526.55) -> (-154.35, 526.55) projected
  line L232 (-154.35, 526.55) -> (-154.35, 525.5) projected
  line L233 (-154.35, 525.5) -> (-157.35, 525.5) projected
  line L234 (-157.35, 525.5) -> (-157.35, 526.55) projected
  line L235 (-157.35, 526.55) -> (-158.65, 526.55) projected
  line L236 (-158.65, 526.55) -> (-158.65, 529) projected
  line L237 (-158.65, 529) -> (-157.35, 529) projected
  line L238 (-157.35, 529) -> (-157.35, 534) projected
  line L239 (-157.35, 534) -> (-195, 534) projected
  line L240 (-195, 534) -> (-195, 26) projected
  line L241 (-195, 26) -> (-145, 26) projected
  line L242 (-145, 26) -> (-145, 324) projected
  line L243 (-145, 324) -> (-125, 344) projected
  line L244 (-125, 344) -> (125, 344) projected
  line L245 (125, 344) -> (145, 324) projected
  line L246 (145, 324) -> (145, 26) projected
  line L247 (145, 26) -> (195, 26) projected
  line L248 (195, 26) -> (195, 534) projected
  line L249 (195, 534) -> (157.35, 534) projected
  line L250 (157.35, 534) -> (157.35, 529) projected
  line L251 (157.35, 529) -> (158.65, 529) projected
  line L252 (158.65, 529) -> (158.65, 526.55) projected
  line L253 (158.65, 526.55) -> (157.35, 526.55) projected
  line L254 (157.35, 526.55) -> (157.35, 525.5) projected
  line L255 (157.35, 525.5) -> (154.35, 525.5) projected
  line L256 (154.35, 525.5) -> (154.35, 526.55) projected
  line L257 (154.35, 526.55) -> (153.05, 526.55) projected
  line L258 (153.05, 526.55) -> (153.05, 529) projected
  line L259 (153.05, 529) -> (154.35, 529) projected
  line L260 (154.35, 529) -> (154.35, 534) projected
  line L261 (154.35, 534) -> (116.7, 534) projected
  line L262 (116.7, 534) -> (116.7, 538) projected
  line L263 (116.7, 538) -> (39.3, 538) projected
  line L264 (39.3, 538) -> (39.3, 534) projected
  line L265 (39.3, 534) -> (1.5, 534) projected
  circle A63 centre (181, 376) radius 5 projected
  circle A64 centre (-181, 376) radius 5 projected
  circle A65 centre (-179, 349) radius 5 projected
  circle A66 centre (179, 349) radius 5 projected
  line L266 (-131.1498, 477.7505) -> (-131.1498, 487.2505) projected
  arc A67 (-130.8998, 487.5005) -> (-131.1498, 487.2505) centre (-130.8998, 487.2505) ccw projected
  line L267 (-130.8998, 487.5005) -> (-108.8998, 487.5005) projected
  arc A68 (-108.6498, 487.2505) -> (-108.8998, 487.5005) centre (-108.8998, 487.2505) ccw projected
  line L268 (-108.6498, 487.2505) -> (-108.6498, 477.7505) projected
  arc A69 (-108.8998, 477.5005) -> (-108.6498, 477.7505) centre (-108.8998, 477.7505) ccw projected
  line L269 (-108.8998, 477.5005) -> (-130.8998, 477.5005) projected
  arc A70 (-131.1498, 477.7505) -> (-130.8998, 477.5005) centre (-130.8998, 477.7505) ccw projected
  spline S95 degree 2 poles (-108.6858, 451.2309) (-108.6858, 452.7138) (-109.7069, 454.8289) (-110.7523, 455.4245) knots 0 0 0 1 2 2 2 projected
  spline S96 degree 2 poles (-110.7523, 455.4245) (-111.5181, 455.8378) (-113.1955, 455.9229) (-114.3625, 455.9229) knots 0 0 0 1 2 2 2 projected
  line L270 (-114.3625, 455.9229) -> (-118.2036, 455.9229) projected
  line L271 (-118.2036, 455.9229) -> (-118.2036, 458.7187) projected
  line L272 (-118.2036, 458.7187) -> (-113.5602, 458.7187) projected
  spline S97 degree 2 poles (-113.5602, 458.7187) (-111.98, 458.7187) (-109.2207, 458.3176) (-108.0051, 457.5396) knots 0 0 0 1 2 2 2 projected
  spline S98 degree 2 poles (-108.0051, 457.5396) (-106.5343, 456.5915) (-104.8203, 453.3825) (-104.8203, 451.2066) knots 0 0 0 1 2 2 2 projected
  spline S99 degree 2 poles (-104.8203, 451.2066) (-104.8203, 449.1036) (-106.6558, 445.7973) (-108.0537, 444.91) knots 0 0 0 1 2 2 2 projected
  spline S100 degree 2 poles (-108.0537, 444.91) (-109.2206, 444.1563) (-111.9678, 443.7186) (-113.5116, 443.7187) knots 0 0 0 1 2 2 2 projected
  line L273 (-113.5116, 443.7187) -> (-118.2036, 443.7187) projected
  line L274 (-118.2036, 443.7187) -> (-118.2036, 446.5267) projected
  line L275 (-118.2036, 446.5267) -> (-114.3625, 446.5267) projected
  spline S101 degree 2 poles (-114.3625, 446.5267) (-113.0983, 446.5267) (-111.36, 446.6118) (-110.5699, 447.1101) knots 0 0 0 1 2 2 2 projected
  spline S102 degree 2 poles (-110.5699, 447.1101) (-109.6461, 447.6936) (-108.6858, 449.7479) (-108.6858, 451.2309) knots 0 0 0 1 2 2 2 projected
  line L276 (-122.3998, 476.0005) -> (-122.3998, 477.0005) projected
  line L277 (-122.3998, 477.0005) -> (-117.3998, 477.0005) projected
  line L278 (-117.3998, 477.0005) -> (-117.3998, 476.0005) projected
  line L279 (-117.3998, 476.0005) -> (-115.3998, 476.0005) projected
  line L280 (-115.3998, 476.0005) -> (-115.3998, 473.0005) projected
  spline S103 degree 2 poles (-115.3998, 473.0005) (-116.5248, 471.7942) (-117.6498, 473.0005) knots -0.936411 -0.936411 -0.936411 0 0 0 weights 1 1.154701 1 projected
  spline S104 degree 2 poles (-117.6498, 473.0005) (-119.8998, 471.7942) (-122.1498, 473.0005) knots -0.936411 -0.936411 -0.936411 0 0 0 weights 1 1.154701 1 projected
  spline S105 degree 2 poles (-122.1498, 473.0005) (-123.2748, 471.7942) (-124.3998, 473.0005) knots 0 0 0 0.936411 0.936411 0.936411 weights 1 1.154701 1 projected
  line L281 (-124.3998, 473.0005) -> (-124.3998, 476.0005) projected
  line L282 (-124.3998, 476.0005) -> (-122.3998, 476.0005) projected
  line L283 (-119.5248, 468.5774) -> (-120.2748, 468.5774) projected
  line L284 (-120.2748, 468.5774) -> (-123.3048, 471.8264) projected
  spline S106 degree 3 poles (-123.3048, 471.8264) (-123.2674, 471.8256) (-123.1923, 471.8269) (-123.099, 471.836) (-123.0063, 471.8503) (-122.9329, 471.866) (-122.8423, 471.8907) (-122.7708, 471.9142) (-122.6828, 471.9483) (-122.6134, 471.9792) (-122.528, 472.0219) (-122.4606, 472.0595) (-122.3773, 472.1105) (-122.3114, 472.1544) (-122.2297, 472.2133) (-122.1486, 472.2762) (-122.0839, 472.3308) (-122.0515, 472.3592) knots 0.459691 0.459691 0.459691 0.459691 0.491589 0.523488 0.539437 0.571336 0.587285 0.619184 0.635133 0.667032 0.682981 0.71488 0.730829 0.762728 0.778677 0.810576 0.842474 0.842474 0.842474 0.842474 projected
  spline S107 degree 3 poles (-122.0515, 472.3592) (-121.923, 472.2982) (-121.6714, 472.1878) (-121.3667, 472.0767) (-121.0671, 471.9849) (-120.8308, 471.9266) (-120.538, 471.872) (-120.3054, 471.843) (-120.0156, 471.8248) (-119.7841, 471.8248) (-119.4942, 471.843) (-119.2616, 471.872) (-118.9103, 471.9375) (-118.4363, 472.064) (-118.0051, 472.2371) (-117.7481, 472.3592) knots 0.060134 0.060134 0.060134 0.060134 0.128146 0.196158 0.230164 0.298176 0.332182 0.400194 0.4342 0.502211 0.536217 0.604229 0.638235 0.740253 0.876277 0.876277 0.876277 0.876277 projected
  spline S108 degree 3 poles (-117.7481, 472.3592) (-117.7158, 472.3308) (-117.6511, 472.2762) (-117.5699, 472.2133) (-117.4882, 472.1544) (-117.4223, 472.1105) (-117.3391, 472.0595) (-117.2717, 472.0219) (-117.1862, 471.9792) (-117.1169, 471.9483) (-117.0288, 471.9142) (-116.9573, 471.8907) (-116.8667, 471.866) (-116.7933, 471.8503) (-116.7007, 471.836) (-116.6073, 471.8269) (-116.5323, 471.8256) (-116.4948, 471.8264) knots 0.093937 0.093937 0.093937 0.093937 0.125835 0.157734 0.173683 0.205582 0.221531 0.25343 0.269379 0.301278 0.317227 0.349126 0.365075 0.396974 0.412923 0.444822 0.47672 0.47672 0.47672 0.47672 projected
  line L285 (-116.4948, 471.8264) -> (-119.5248, 468.5774) projected
  line L286 (-114.4354, 446.5678) -> (-118.2036, 446.5678) projected
  line L287 (-118.2036, 446.5678) -> (-118.2036, 455.9186) projected
  line L288 (-118.2036, 455.9186) -> (-114.4354, 455.9186) projected
  line L289 (-114.4354, 455.9186) -> (-114.4354, 446.5678) projected
  arc A71 (-119.3998, 461.3273) -> (-120.8998, 462.8273) centre (-120.8998, 461.3273) ccw projected
  line L290 (-119.3998, 461.3273) -> (-119.3998, 460.8273) projected
  line L291 (-119.3998, 460.8273) -> (-120.3998, 460.8273) projected
  line L292 (-120.3998, 460.8273) -> (-120.3998, 461.3273) projected
  arc A72 (-120.3998, 461.3273) -> (-120.8998, 461.8273) centre (-120.8998, 461.3273) ccw projected
  line L293 (-120.8998, 461.8273) -> (-127.3998, 461.8273) projected
  arc A73 (-127.3998, 464.8273) -> (-127.3998, 461.8273) centre (-127.3998, 463.3273) ccw projected
  line L294 (-127.3998, 464.8273) -> (-112.3998, 464.8273) projected
  arc A74 (-112.3998, 464.8273) -> (-112.3998, 465.8273) centre (-112.3998, 465.3273) ccw projected
  line L295 (-112.3998, 465.8273) -> (-118.8998, 465.8273) projected
  arc A75 (-120.3998, 467.3273) -> (-118.8998, 465.8273) centre (-118.8998, 467.3273) ccw projected
  line L296 (-120.3998, 467.3273) -> (-120.3998, 467.8273) projected
  line L297 (-120.3998, 467.8273) -> (-119.3998, 467.8273) projected
  line L298 (-119.3998, 467.8273) -> (-119.3998, 467.3273) projected
  arc A76 (-119.3998, 467.3273) -> (-118.8998, 466.8273) centre (-118.8998, 467.3273) ccw projected
  line L299 (-118.8998, 466.8273) -> (-112.3998, 466.8273) projected
  arc A77 (-112.3998, 463.8273) -> (-112.3998, 466.8273) centre (-112.3998, 465.3273) ccw projected
  line L300 (-112.3998, 463.8273) -> (-127.3998, 463.8273) projected
  arc A78 (-127.3998, 463.8273) -> (-127.3998, 462.8273) centre (-127.3998, 463.3273) ccw projected
  line L301 (-127.3998, 462.8273) -> (-120.8998, 462.8273) projected
  spline S109 degree 2 poles (-122.6526, 458.1231) (-121.8868, 457.649) (-121.121, 456.1904) (-121.121, 455.2787) knots 0 0 0 1 2 2 2 projected
  spline S110 degree 2 poles (-121.121, 455.2787) (-121.121, 453.9902) (-122.604, 452.0696) (-123.8195, 451.79) knots 0 0 0 1 2 2 2 projected
  line L302 (-123.8195, 451.79) -> (-123.8195, 451.6442) projected
  spline S111 degree 2 poles (-123.8195, 451.6442) (-123.2847, 451.5712) (-122.2636, 451.1822) (-121.7774, 450.7446) knots 0 0 0 1 2 2 2 projected
  spline S112 degree 2 poles (-121.7774, 450.7446) (-121.3276, 450.3557) (-120.732, 449.1158) (-120.732, 448.2649) knots 0 0 0 1 2 2 2 projected
  spline S113 degree 2 poles (-120.732, 448.2649) (-120.732, 447.1587) (-121.5464, 445.3476) (-122.3365, 444.7155) knots 0 0 0 1 2 2 2 projected
  spline S114 degree 2 poles (-122.3365, 444.7155) (-123.1267, 444.0834) (-125.2782, 443.4027) (-126.822, 443.4027) knots 0 0 0 1 2 2 2 projected
  spline S115 degree 2 poles (-126.822, 443.4027) (-128.5724, 443.4026) (-131.0764, 443.9861) (-131.8665, 444.3508) knots 0 0 0 1 2 2 2 projected
  line L303 (-131.8665, 444.3508) -> (-131.8665, 447.6085) projected
  line L304 (-131.8665, 447.6085) -> (-131.5019, 447.6085) projected
  spline S116 degree 2 poles (-131.5019, 447.6085) (-130.6753, 447.0858) (-128.4508, 446.3079) (-127.527, 446.3079) knots 0 0 0 1 2 2 2 projected
  spline S117 degree 2 poles (-127.527, 446.3079) (-126.98, 446.3079) (-125.7036, 446.5024) (-125.266, 446.8184) knots 0 0 0 1 2 2 2 projected
  spline S118 degree 2 poles (-125.266, 446.8184) (-124.9257, 447.0737) (-124.5124, 447.8151) (-124.5124, 448.4837) knots 0 0 0 1 2 2 2 projected
  spline S119 degree 2 poles (-124.5124, 448.4837) (-124.5124, 449.1523) (-125.0959, 449.8694) (-125.5821, 450.0396) knots 0 0 0 1 2 2 2 projected
  spline S120 degree 2 poles (-125.5821, 450.0396) (-126.0683, 450.2098) (-127.4176, 450.2463) (-127.9403, 450.2463) knots 0 0 0 1 2 2 2 projected
  line L305 (-127.9403, 450.2463) -> (-128.5845, 450.2463) projected
  line L306 (-128.5845, 450.2463) -> (-128.5845, 452.884) projected
  line L307 (-128.5845, 452.884) -> (-127.9889, 452.884) projected
  spline S121 degree 2 poles (-127.9889, 452.884) (-127.3082, 452.884) (-126.1534, 453.0056) (-125.7523, 453.1879) knots 0 0 0 1 2 2 2 projected
  spline S122 degree 2 poles (-125.7523, 453.1879) (-125.3511, 453.3824) (-124.9014, 454.0631) (-124.9014, 454.6466) knots 0 0 0 1 2 2 2 projected
  spline S123 degree 2 poles (-124.9014, 454.6466) (-124.9014, 455.1085) (-125.3268, 455.6798) (-125.6307, 455.8378) knots 0 0 0 1 2 2 2 projected
  spline S124 degree 2 poles (-125.6307, 455.8378) (-125.9954, 456.0202) (-126.9678, 456.1417) (-127.3082, 456.1417) knots 0 0 0 1 2 2 2 projected
  spline S125 degree 2 poles (-127.3082, 456.1417) (-127.8552, 456.1417) (-129.01, 455.8864) (-129.5448, 455.6798) knots 0 0 0 1 2 2 2 projected
  spline S126 degree 2 poles (-129.5448, 455.6798) (-129.9703, 455.5218) (-130.7084, 455.1139) (-130.8976, 455.0047) knots 0 0 0 1 1.597943 1.597943 1.597943 projected
  line L308 (-130.8976, 455.0047) -> (-131.3629, 454.8775) projected
  line L309 (-131.3629, 454.8775) -> (-131.4289, 454.8775) projected
  line L310 (-131.4289, 454.8775) -> (-131.4289, 458.0866) projected
  spline S127 degree 2 poles (-131.4289, 458.0866) (-130.651, 458.4148) (-128.0254, 459.0348) (-126.6518, 459.0348) knots 0 0 0 1 2 2 2 projected
  spline S128 degree 2 poles (-126.6518, 459.0348) (-125.3147, 459.0348) (-123.3455, 458.5729) (-122.6526, 458.1231) knots 0 0 0 1 2 2 2 projected
  line L311 (-119.9951, 430.5006) -> (-119.9951, 437.0006) projected
  arc A79 (-119.9951, 437.0006) -> (-119.9952, 437.0006) centre (-119.8998, 464.5005) ccw projected
  line L312 (-119.9952, 437.0006) -> (-119.9952, 430.5006) projected
  arc A80 (-124.3998, 430.7996) -> (-119.9952, 430.5006) centre (-119.8998, 464.5005) ccw projected
  arc A81 (-126.1498, 434.137) -> (-124.3998, 430.7996) centre (-112.6193, 439.1042) ccw projected
  arc A82 (-136.9506, 438.6109) -> (-126.1498, 434.137) centre (-119.8998, 464.5005) ccw projected
  arc A83 (-140.548, 437.4884) -> (-136.9506, 438.6109) centre (-143.0058, 451.6907) ccw projected
  arc A84 (-146.9119, 443.8523) -> (-140.548, 437.4884) centre (-119.8998, 464.5005) ccw projected
  arc A85 (-145.7894, 447.4497) -> (-146.9119, 443.8523) centre (-132.7096, 441.3945) ccw projected
  arc A86 (-150.2632, 458.2505) -> (-145.7894, 447.4497) centre (-119.8998, 464.5005) ccw projected
  arc A87 (-153.6007, 460.0005) -> (-150.2632, 458.2505) centre (-145.2961, 471.781) ccw projected
  arc A88 (-153.6007, 469.0005) -> (-153.6007, 460.0005) centre (-119.8998, 464.5005) ccw projected
  arc A89 (-150.2632, 470.7505) -> (-153.6007, 469.0005) centre (-145.2961, 457.2199) ccw projected
  arc A90 (-145.7894, 481.5512) -> (-150.2632, 470.7505) centre (-119.8998, 464.5005) ccw projected
  arc A91 (-146.9119, 485.1486) -> (-145.7894, 481.5512) centre (-132.7096, 487.6064) ccw projected
  arc A92 (-140.548, 491.5126) -> (-146.9119, 485.1486) centre (-119.8998, 464.5005) ccw projected
  arc A93 (-136.9506, 490.3901) -> (-140.548, 491.5126) centre (-143.0058, 477.3102) ccw projected
  arc A94 (-126.1498, 494.8639) -> (-136.9506, 490.3901) centre (-119.8998, 464.5005) ccw projected
  arc A95 (-124.3998, 498.2014) -> (-126.1498, 494.8639) centre (-112.6193, 489.8967) ccw projected
  arc A96 (-115.3998, 498.2014) -> (-124.3998, 498.2014) centre (-119.8998, 464.5005) ccw projected
  arc A97 (-113.6498, 494.8639) -> (-115.3998, 498.2014) centre (-127.1803, 489.8967) ccw projected
  arc A98 (-102.8491, 490.3901) -> (-113.6498, 494.8639) centre (-119.8998, 464.5005) ccw projected
  arc A99 (-99.2517, 491.5126) -> (-102.8491, 490.3901) centre (-96.7939, 477.3102) ccw projected
  arc A100 (-92.8877, 485.1486) -> (-99.2517, 491.5126) centre (-119.8998, 464.5005) ccw projected
  arc A101 (-94.0102, 481.5512) -> (-92.8877, 485.1486) centre (-107.0901, 487.6064) ccw projected
  arc A102 (-89.5364, 470.7505) -> (-94.0102, 481.5512) centre (-119.8998, 464.5005) ccw projected
  arc A103 (-86.1989, 469.0005) -> (-89.5364, 470.7505) centre (-94.5036, 457.2199) ccw projected
  arc A104 (-86.1989, 460.0005) -> (-86.1989, 469.0005) centre (-119.8998, 464.5005) ccw projected
  arc A105 (-89.5364, 458.2505) -> (-86.1989, 460.0005) centre (-94.5036, 471.781) ccw projected
  arc A106 (-94.0102, 447.4497) -> (-89.5364, 458.2505) centre (-119.8998, 464.5005) ccw projected
  arc A107 (-92.8877, 443.8523) -> (-94.0102, 447.4497) centre (-107.0901, 441.3945) ccw projected
  arc A108 (-99.2517, 437.4884) -> (-92.8877, 443.8523) centre (-119.8998, 464.5005) ccw projected
  arc A109 (-102.8491, 438.6109) -> (-99.2517, 437.4884) centre (-96.7939, 451.6907) ccw projected
  arc A110 (-113.6498, 434.137) -> (-102.8491, 438.6109) centre (-119.8998, 464.5005) ccw projected
  arc A111 (-115.3998, 430.7996) -> (-113.6498, 434.137) centre (-127.1803, 439.1042) ccw projected
  arc A112 (-119.9951, 430.5006) -> (-115.3998, 430.7996) centre (-119.8998, 464.5005) ccw projected
  circle A113 centre (1, 464) radius 20.6 projected
  circle A114 centre (179.5, 40) radius 2 projected
  circle A115 centre (-179.5, 79.5) radius 2 projected
  circle A116 centre (-179.5, 337) radius 2 projected
  circle A117 centre (179.5, 337) radius 2 projected
  circle A118 centre (179.5, 255) radius 2.875 projected
  circle A119 centre (-179.5, 308) radius 2 projected
  circle A120 centre (-179.5, 40) radius 2 projected
  circle A121 centre (-158.75, 122) radius 1.5 projected
  circle A122 centre (-158.75, 254) radius 1.5 projected
  circle A123 centre (-158.75, 284) radius 1.5 projected
  circle A124 centre (-158.75, 92) radius 1.5 projected
  circle A125 centre (150.2671, 178.4783) radius 1.5 projected
  line L313 (116.2244, 383.4424) -> (116.2244, 380.5646) projected
  line L314 (116.2244, 380.5646) -> (110.4314, 380.5646) projected
  line L315 (110.4314, 380.5646) -> (110.1311, 378.6127) projected
  spline S129 degree 2 poles (110.1311, 378.6127) (110.7316, 378.888) (111.9078, 379.1758) (112.4833, 379.1758) knots 0 0 0 1 2 2 2 projected
  spline S130 degree 2 poles (112.4833, 379.1758) (114.4227, 379.1758) (116.85, 376.811) (116.85, 375.0218) knots 0 0 0 1 2 2 2 projected
  spline S131 degree 2 poles (116.85, 375.0218) (116.85, 373.7706) (115.5988, 371.4433) (113.3091, 370.2172) (111.5199, 370.2172) knots 0 0 0 1 2 3 3 3 projected
  spline S132 degree 2 poles (111.5199, 370.2172) (110.2312, 370.2172) (108.4044, 370.7051) (107.1157, 371.6686) (106.3149, 372.8947) (106.0521, 373.8081) knots 0 0 0 1 2 3 4 4 4 projected
  line L316 (106.0521, 373.8081) -> (109.7057, 374.2085) projected
  spline S133 degree 2 poles (109.7057, 374.2085) (109.8433, 373.3327) (110.8067, 372.4193) (111.4824, 372.4193) knots 0 0 0 1 2 2 2 projected
  spline S134 degree 2 poles (111.4824, 372.4193) (112.2331, 372.4193) (113.209, 373.5579) (113.209, 374.6965) knots 0 0 0 1 2 2 2 projected
  spline S135 degree 2 poles (113.209, 374.6965) (113.209, 375.8601) (112.2206, 376.9361) (111.4073, 376.9361) knots 0 0 0 1 2 2 2 projected
  spline S136 degree 2 poles (111.4073, 376.9361) (110.8818, 376.9361) (110.3938, 376.6734) knots 0 0 0 1 1 1 projected
  spline S137 degree 2 poles (110.3938, 376.6734) (110.0435, 376.4982) (109.6056, 376.0102) knots 0 0 0 1 1 1 projected
  line L317 (109.6056, 376.0102) -> (106.5276, 376.4481) projected
  line L318 (106.5276, 376.4481) -> (107.6662, 383.4424) projected
  line L319 (107.6662, 383.4424) -> (116.2244, 383.4424) projected
  spline S138 degree 2 poles (77.5998, 374.9842) (77.7249, 374.0458) (78.1003, 373.5579) knots 0 0 0 1 1 1 projected
  spline S139 degree 2 poles (78.1003, 373.5579) (78.7259, 372.7696) (79.8895, 372.7696) knots 0 0 0 1 1 1 projected
  spline S140 degree 2 poles (79.8895, 372.7696) (80.7403, 372.7696) (81.6787, 373.5829) (81.6787, 374.1084) knots 0 0 0 1 2 2 2 projected
  spline S141 degree 2 poles (81.6787, 374.1084) (81.6787, 374.6089) (81.2283, 375.0093) knots 0 0 0 1 1 1 projected
  spline S142 degree 2 poles (81.2283, 375.0093) (80.7904, 375.4096) (79.1763, 375.7725) knots 0 0 0 1 1 1 projected
  spline S143 degree 2 poles (79.1763, 375.7725) (76.5237, 376.3606) (75.3977, 377.349) knots 0 0 0 1 1 1 projected
  spline S144 degree 2 poles (75.3977, 377.349) (74.2591, 378.3375) (74.2591, 379.8639) knots 0 0 0 1 1 1 projected
  spline S145 degree 2 poles (74.2591, 379.8639) (74.2591, 380.8649) (75.4227, 382.6416) (77.7624, 383.6676) (79.7894, 383.6676) knots 0 0 0 1 2 3 3 3 projected
  spline S146 degree 2 poles (79.7894, 383.6676) (82.2918, 383.6676) (84.9068, 381.8158) (85.157, 379.7889) knots 0 0 0 1 2 2 2 projected
  line L320 (85.157, 379.7889) -> (81.3659, 379.5636) projected
  spline S147 degree 2 poles (81.3659, 379.5636) (81.2158, 380.4395) (80.2398, 381.2403) (79.389, 381.2403) knots 0 0 0 1 2 2 2 projected
  spline S148 degree 2 poles (79.389, 381.2403) (78.6883, 381.2403) (77.9751, 380.6522) (77.9751, 380.2143) knots 0 0 0 1 2 2 2 projected
  spline S149 degree 2 poles (77.9751, 380.2143) (77.9751, 379.914) (78.2754, 379.6637) knots 0 0 0 1 1 1 projected
  spline S150 degree 2 poles (78.2754, 379.6637) (78.5632, 379.401) (79.6267, 379.1883) knots 0 0 0 1 1 1 projected
  spline S151 degree 2 poles (79.6267, 379.1883) (82.2668, 378.6127) (84.544, 377.4491) (85.5825, 375.735) (85.5825, 374.6714) knots 0 0 0 1 2 3 3 3 projected